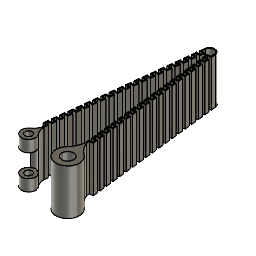
bones_v1 (Autodesk Fusion 360 design; units mm, degrees)
Autodesk Fusion 360 part; units mm, degrees
sketch "Sketch1" plane through (0, 0, 0) normal (0, 0, 1) x (1, 0, 0)
  circle A0 centre (68.7652, 38.9351) radius 1.9
  circle A1 centre (68.7652, 38.9351) radius 3.775
  line L0 (68.7652, 38.9351) -> (89.7652, 38.9351) construction
  circle A2 centre (89.7652, 38.9351) radius 3.175
  circle A3 centre (89.7652, 38.9351) radius 6.35
  line L1 (79.2652, 131.0925) -> (89.7652, 38.9351) construction
  line L2 (79.2652, 131.0925) -> (68.7652, 38.9351) construction
  line L3 (89.0463, 45.2443) -> (88.4803, 50.2122) construction
  line L4 (88.4803, 50.2122) -> (88.7287, 50.2405)
  line L5 (88.4803, 50.2122) -> (88.2319, 50.1839)
  line L6 (88.2319, 50.1839) -> (88.0055, 52.171)
  line L7 (88.7287, 50.2405) -> (88.5589, 51.7308)
  line L8 (88.0055, 52.171) -> (89.9927, 52.3974)
  line L9 (88.5589, 51.7308) -> (90.5461, 51.9573)
  line L10 (89.9927, 52.3974) -> (89.8229, 53.8878)
  line L11 (90.5461, 51.9573) -> (90.2631, 54.4412)
  line L12 (89.8229, 53.8878) -> (87.8357, 53.6614)
  line L13 (90.2631, 54.4412) -> (88.2759, 54.2148)
  line L14 (87.8357, 53.6614) -> (87.5527, 56.1453)
  line L15 (88.2759, 54.2148) -> (88.1061, 55.7051)
  line L16 (89.2261, 43.667) -> (93.3992, 44.1425) construction
  line L17 (89.2261, 43.667) -> (85.0529, 43.1916) construction
  arc A4 (85.0529, 43.1916) -> (88.2319, 50.1839) centre (75.649, 51.6858) ccw
  arc A5 (88.7287, 50.2405) -> (93.3992, 44.1425) centre (100.6513, 54.5345) ccw
  line L18 (88.1061, 55.7051) -> (90.0933, 55.9315)
  line L19 (87.5527, 56.1453) -> (89.5399, 56.3717)
  line L20 (89.5399, 56.3717) -> (89.3701, 57.8621)
  line L21 (90.0933, 55.9315) -> (89.8102, 58.4155)
  line L22 (89.8102, 58.4155) -> (87.8231, 58.1891)
  line L23 (89.3701, 57.8621) -> (87.3829, 57.6357)
  line L24 (87.3829, 57.6357) -> (87.0999, 60.1196)
  line L25 (87.8231, 58.1891) -> (87.6533, 59.6794)
  line L26 (87.6533, 59.6794) -> (89.6404, 59.9058)
  line L27 (87.0999, 60.1196) -> (89.0871, 60.346)
  line L28 (89.0871, 60.346) -> (88.9172, 61.8364)
  line L29 (89.6404, 59.9058) -> (89.3574, 62.3898)
  line L30 (88.9172, 61.8364) -> (86.9301, 61.61)
  line L31 (89.3574, 62.3898) -> (87.3703, 62.1634)
  line L32 (86.9301, 61.61) -> (86.6471, 64.0939)
  line L33 (87.3703, 62.1634) -> (87.2005, 63.6537)
  line L34 (87.2005, 63.6537) -> (89.1876, 63.8801)
  line L35 (86.6471, 64.0939) -> (88.6342, 64.3203)
  line L36 (88.6342, 64.3203) -> (88.4644, 65.8107)
  line L37 (89.1876, 63.8801) -> (88.9046, 66.364)
  line L38 (88.4644, 65.8107) -> (86.4773, 65.5843)
  line L39 (88.9046, 66.364) -> (86.9175, 66.1376)
  line L40 (86.4773, 65.5843) -> (86.1943, 68.0682)
  line L41 (86.9175, 66.1376) -> (86.7477, 67.628)
  line L42 (86.7477, 67.628) -> (88.7348, 67.8544)
  line L43 (86.1943, 68.0682) -> (88.1814, 68.2946)
  line L44 (88.1814, 68.2946) -> (88.0116, 69.7849)
  line L45 (88.7348, 67.8544) -> (88.4518, 70.3383)
  line L46 (88.0116, 69.7849) -> (86.0245, 69.5585)
  line L47 (88.4518, 70.3383) -> (86.4647, 70.1119)
  line L48 (86.0245, 69.5585) -> (85.7415, 72.0425)
  line L49 (86.4647, 70.1119) -> (86.2949, 71.6023)
  line L50 (86.2949, 71.6023) -> (88.282, 71.8287)
  line L51 (85.7415, 72.0425) -> (87.7286, 72.2689)
  line L52 (87.7286, 72.2689) -> (87.5588, 73.7592)
  line L53 (88.282, 71.8287) -> (87.999, 74.3126)
  line L54 (87.5588, 73.7592) -> (85.5717, 73.5328)
  line L55 (87.999, 74.3126) -> (86.0118, 74.0862)
  line L56 (85.5717, 73.5328) -> (85.2887, 76.0168)
  line L57 (86.0118, 74.0862) -> (85.842, 75.5766)
  line L58 (85.842, 75.5766) -> (87.8292, 75.803)
  line L59 (85.2887, 76.0168) -> (87.2758, 76.2432)
  line L60 (87.2758, 76.2432) -> (87.106, 77.7335)
  line L61 (87.8292, 75.803) -> (87.5462, 78.2869)
  line L62 (87.106, 77.7335) -> (85.1189, 77.5071)
  line L63 (87.5462, 78.2869) -> (85.559, 78.0605)
  line L64 (85.1189, 77.5071) -> (84.8358, 79.991)
  line L65 (85.559, 78.0605) -> (85.3892, 79.5509)
  line L66 (85.3892, 79.5509) -> (87.3764, 79.7773)
  line L67 (84.8358, 79.991) -> (86.823, 80.2175)
  line L68 (86.823, 80.2175) -> (86.6532, 81.7078)
  line L69 (87.3764, 79.7773) -> (87.0934, 82.2612)
  line L70 (86.6532, 81.7078) -> (84.666, 81.4814)
  line L71 (87.0934, 82.2612) -> (85.1062, 82.0348)
  line L72 (84.666, 81.4814) -> (84.383, 83.9653)
  line L73 (85.1062, 82.0348) -> (84.9364, 83.5251)
  line L74 (84.9364, 83.5251) -> (86.9236, 83.7516)
  line L75 (84.383, 83.9653) -> (86.3702, 84.1917)
  line L76 (86.3702, 84.1917) -> (86.2004, 85.6821)
  line L77 (86.9236, 83.7516) -> (86.6406, 86.2355)
  line L78 (86.2004, 85.6821) -> (84.2132, 85.4557)
  line L79 (86.6406, 86.2355) -> (84.6534, 86.0091)
  line L80 (84.2132, 85.4557) -> (83.9302, 87.9396)
  line L81 (84.6534, 86.0091) -> (84.4836, 87.4994)
  line L82 (84.4836, 87.4994) -> (86.4707, 87.7258)
  line L83 (83.9302, 87.9396) -> (85.9174, 88.166)
  line L84 (85.9174, 88.166) -> (85.7476, 89.6564)
  line L85 (86.4707, 87.7258) -> (86.1877, 90.2098)
  line L86 (85.7476, 89.6564) -> (83.7604, 89.43)
  line L87 (86.1877, 90.2098) -> (84.2006, 89.9834)
  line L88 (83.7604, 89.43) -> (83.4774, 91.9139)
  line L89 (84.2006, 89.9834) -> (84.0308, 91.4737)
  line L90 (84.0308, 91.4737) -> (86.0179, 91.7001)
  line L91 (83.4774, 91.9139) -> (85.4645, 92.1403)
  line L92 (85.4645, 92.1403) -> (85.2947, 93.6307)
  line L93 (86.0179, 91.7001) -> (85.7349, 94.1841)
  line L94 (85.2947, 93.6307) -> (83.3076, 93.4043)
  line L95 (85.7349, 94.1841) -> (83.7478, 93.9577)
  line L96 (83.3076, 93.4043) -> (83.0246, 95.8882)
  line L97 (83.7478, 93.9577) -> (83.578, 95.448)
  line L98 (83.578, 95.448) -> (85.5651, 95.6744)
  line L99 (83.0246, 95.8882) -> (85.0117, 96.1146)
  line L100 (85.0117, 96.1146) -> (84.8419, 97.605)
  line L101 (85.5651, 95.6744) -> (85.2821, 98.1583)
  line L102 (84.8419, 97.605) -> (82.8548, 97.3786)
  line L103 (85.2821, 98.1583) -> (83.295, 97.9319)
  line L104 (82.8548, 97.3786) -> (82.5718, 99.8625)
  line L105 (83.295, 97.9319) -> (83.1252, 99.4223)
  line L106 (83.1252, 99.4223) -> (85.1123, 99.6487)
  line L107 (82.5718, 99.8625) -> (84.5589, 100.0889)
  line L108 (84.5589, 100.0889) -> (84.3891, 101.5792)
  line L109 (85.1123, 99.6487) -> (84.8293, 102.1326)
  line L110 (84.3891, 101.5792) -> (82.402, 101.3528)
  line L111 (84.8293, 102.1326) -> (82.8422, 101.9062)
  line L112 (82.402, 101.3528) -> (82.119, 103.8368)
  line L113 (82.8422, 101.9062) -> (82.6724, 103.3966)
  line L114 (82.6724, 103.3966) -> (84.6595, 103.623)
  line L115 (82.119, 103.8368) -> (84.1061, 104.0632)
  line L116 (84.1061, 104.0632) -> (83.9363, 105.5535)
  line L117 (84.6595, 103.623) -> (84.3765, 106.1069)
  line L118 (83.9363, 105.5535) -> (81.9492, 105.3271)
  line L119 (84.3765, 106.1069) -> (82.3893, 105.8805)
  line L120 (81.9492, 105.3271) -> (81.6662, 107.8111)
  line L121 (82.3893, 105.8805) -> (82.2195, 107.3709)
  line L122 (82.2195, 107.3709) -> (84.2067, 107.5973)
  line L123 (81.6662, 107.8111) -> (83.6533, 108.0375)
  line L124 (83.6533, 108.0375) -> (83.4835, 109.5278)
  line L125 (84.2067, 107.5973) -> (83.9237, 110.0812)
  line L126 (83.4835, 109.5278) -> (81.4963, 109.3014)
  line L127 (83.9237, 110.0812) -> (81.9365, 109.8548)
  line L128 (81.4963, 109.3014) -> (81.2133, 111.7853)
  line L129 (81.9365, 109.8548) -> (81.7667, 111.3452)
  line L130 (81.7667, 111.3452) -> (83.7539, 111.5716)
  line L131 (81.2133, 111.7853) -> (83.2005, 112.0118)
  line L132 (83.2005, 112.0118) -> (83.0307, 113.5021)
  line L133 (83.7539, 111.5716) -> (83.4709, 114.0555)
  line L134 (83.0307, 113.5021) -> (81.0435, 113.2757)
  line L135 (83.4709, 114.0555) -> (81.4837, 113.8291)
  line L136 (81.0435, 113.2757) -> (80.7605, 115.7596)
  line L137 (81.4837, 113.8291) -> (81.3139, 115.3194)
  line L138 (88.5589, 51.7308) -> (90.5461, 51.9573)
  line L139 (88.0055, 52.171) -> (89.9927, 52.3974)
  line L140 (89.9927, 52.3974) -> (89.8229, 53.8878)
  line L141 (90.5461, 51.9573) -> (90.2631, 54.4412)
  line L142 (89.8229, 53.8878) -> (87.8357, 53.6614)
  line L143 (90.2631, 54.4412) -> (88.2759, 54.2148)
  line L144 (87.8357, 53.6614) -> (87.5527, 56.1453)
  line L145 (88.2759, 54.2148) -> (88.1061, 55.7051)
  line L146 (88.1061, 55.7051) -> (90.0933, 55.9315)
  line L147 (87.5527, 56.1453) -> (89.5399, 56.3717)
  line L148 (89.5399, 56.3717) -> (89.3701, 57.8621)
  line L149 (90.0933, 55.9315) -> (89.8102, 58.4155)
  line L150 (89.3701, 57.8621) -> (87.3829, 57.6357)
  line L151 (89.8102, 58.4155) -> (87.8231, 58.1891)
  line L152 (87.3829, 57.6357) -> (87.0999, 60.1196)
  line L153 (87.8231, 58.1891) -> (87.6533, 59.6794)
  line L154 (81.3139, 115.3194) -> (83.3011, 115.5459)
  line L155 (80.7605, 115.7596) -> (82.7477, 115.986)
  line L156 (82.7477, 115.986) -> (82.5779, 117.4764)
  line L157 (83.3011, 115.5459) -> (83.0181, 118.0298)
  line L158 (82.5779, 117.4764) -> (80.5907, 117.25)
  line L159 (83.0181, 118.0298) -> (81.0309, 117.8034)
  line L160 (80.5907, 117.25) -> (80.3077, 119.7339)
  line L161 (81.0309, 117.8034) -> (80.8611, 119.2937)
  line L162 (80.8611, 119.2937) -> (82.8482, 119.5201)
  line L163 (80.3077, 119.7339) -> (82.2949, 119.9603)
  line L164 (82.2949, 119.9603) -> (82.1251, 121.4507)
  line L165 (82.8482, 119.5201) -> (82.5652, 122.0041)
  line L166 (82.1251, 121.4507) -> (80.1379, 121.2243)
  line L167 (82.5652, 122.0041) -> (80.5781, 121.7777)
  line L168 (80.1379, 121.2243) -> (79.8549, 123.7082)
  line L169 (80.5781, 121.7777) -> (80.4083, 123.268)
  line L170 (80.4083, 123.268) -> (82.3954, 123.4944)
  line L171 (79.8549, 123.7082) -> (81.842, 123.9346)
  line L172 (81.842, 123.9346) -> (81.6722, 125.425)
  line L173 (82.3954, 123.4944) -> (82.1124, 125.9784)
  line L174 (79.2652, 131.0925) -> (79.2652, 38.9351) construction
  line L175 (80.8611, 119.2937) -> (82.8482, 119.5201)
  line L176 (80.3077, 119.7339) -> (82.2949, 119.9603)
  line L177 (82.2949, 119.9603) -> (82.1251, 121.4507)
  line L178 (82.8482, 119.5201) -> (82.5652, 122.0041)
  line L179 (76.141, 105.8805) -> (76.3108, 107.3709)
  line L180 (75.0469, 109.5278) -> (77.034, 109.3014)
  line L181 (74.6067, 110.0812) -> (76.5938, 109.8548)
  line L182 (74.1539, 106.1069) -> (76.141, 105.8805)
  line L183 (73.7011, 102.1326) -> (75.6882, 101.9062)
  line L184 (76.1284, 101.3528) -> (76.4114, 103.8368)
  line L185 (74.5941, 105.5535) -> (76.5812, 105.3271)
  line L186 (74.3237, 107.5973) -> (74.6067, 110.0812)
  line L187 (74.1413, 101.5792) -> (76.1284, 101.3528)
  line L188 (76.5812, 105.3271) -> (76.8642, 107.8111)
  line L189 (73.4181, 99.6487) -> (73.7011, 102.1326)
  line L190 (75.6821, 119.5201) -> (75.9651, 122.0041)
  line L191 (76.6883, 123.9346) -> (76.8581, 125.425)
  line L192 (76.2355, 119.9603) -> (76.4053, 121.4507)
  line L193 (77.9523, 121.7777) -> (78.1221, 123.268)
  line L194 (77.9397, 117.25) -> (78.2227, 119.7339)
  line L195 (77.4868, 113.2757) -> (77.7699, 115.7596)
  line L196 (78.6755, 123.7082) -> (76.6883, 123.9346)
  line L197 (75.5123, 118.0298) -> (77.4995, 117.8034)
  line L198 (70.6946, 53.6614) -> (70.9777, 56.1453)
  line L199 (75.4997, 113.5021) -> (77.4868, 113.2757)
  line L200 (77.0467, 113.8291) -> (77.2165, 115.3194)
  line L201 (78.1221, 123.268) -> (76.1349, 123.4944)
  line L202 (70.6946, 53.6614) -> (70.9777, 56.1453)
  line L203 (74.3172, 85.4557) -> (74.6002, 87.9396)
  line L204 (77.6693, 119.2937) -> (75.6821, 119.5201)
  line L205 (78.3925, 121.2243) -> (78.6755, 123.7082)
  line L206 (75.9651, 122.0041) -> (77.9523, 121.7777)
  line L207 (75.9525, 117.4764) -> (77.9397, 117.25)
  line L208 (70.2545, 54.2148) -> (70.4243, 55.7051)
  line L209 (78.2227, 119.7339) -> (76.2355, 119.9603)
  line L210 (76.4053, 121.4507) -> (78.3925, 121.2243)
  line L211 (70.2545, 54.2148) -> (70.4243, 55.7051)
  line L212 (75.2293, 115.5459) -> (75.5123, 118.0298)
  line L213 (75.0595, 114.0555) -> (77.0467, 113.8291)
  line L214 (76.2355, 119.9603) -> (76.4053, 121.4507)
  line L215 (68.4371, 55.9315) -> (68.7201, 58.4155)
  line L216 (69.9715, 51.7308) -> (67.9843, 51.9573)
  line L217 (77.2165, 115.3194) -> (75.2293, 115.5459)
  line L218 (77.317, 111.7853) -> (75.3299, 112.0118)
  line L219 (70.5248, 52.171) -> (68.5377, 52.3974)
  line L220 (68.7075, 53.8878) -> (70.6946, 53.6614)
  line L221 (75.3299, 112.0118) -> (75.4997, 113.5021)
  line L222 (70.5248, 52.171) -> (68.5377, 52.3974)
  line L223 (76.7636, 111.3452) -> (74.7765, 111.5716)
  line L224 (77.7699, 115.7596) -> (75.7827, 115.986)
  line L225 (68.2673, 54.4412) -> (70.2545, 54.2148)
  line L226 (74.7765, 111.5716) -> (75.0595, 114.0555)
  line L227 (73.5186, 96.1146) -> (73.6884, 97.605)
  line L228 (75.6821, 119.5201) -> (75.9651, 122.0041)
  line L229 (75.7827, 115.986) -> (75.9525, 117.4764)
  line L230 (72.9653, 95.6744) -> (73.2483, 98.1583)
  line L231 (77.034, 109.3014) -> (77.317, 111.7853)
  line L232 (76.5938, 109.8548) -> (76.7636, 111.3452)
  line L233 (68.7075, 53.8878) -> (70.6946, 53.6614)
  line L234 (78.2227, 119.7339) -> (76.2355, 119.9603)
  line L235 (77.4995, 117.8034) -> (77.6693, 119.2937)
  line L236 (68.5377, 52.3974) -> (68.7075, 53.8878)
  line L237 (67.9843, 51.9573) -> (68.2673, 54.4412)
  line L238 (68.2673, 54.4412) -> (70.2545, 54.2148)
  line L239 (77.6693, 119.2937) -> (75.6821, 119.5201)
  line L240 (67.9843, 51.9573) -> (68.2673, 54.4412)
  line L241 (68.5377, 52.3974) -> (68.7075, 53.8878)
  line L242 (76.1349, 123.4944) -> (76.418, 125.9784)
  line L243 (69.9715, 51.7308) -> (67.9843, 51.9573)
  line L244 (68.9905, 56.3717) -> (69.1603, 57.8621)
  line L245 (74.1473, 83.9653) -> (72.1602, 84.1917)
  line L246 (73.594, 83.5251) -> (71.6068, 83.7516)
  line L247 (68.7201, 58.4155) -> (70.7073, 58.1891)
  line L248 (73.2417, 76.0168) -> (71.2546, 76.2432)
  line L249 (69.1603, 57.8621) -> (71.1475, 57.6357)
  line L250 (70.4243, 55.7051) -> (68.4371, 55.9315)
  line L251 (70.9777, 56.1453) -> (68.9905, 56.3717)
  line L252 (71.154, 79.7773) -> (71.437, 82.2612)
  line L253 (73.4115, 77.5071) -> (73.6945, 79.991)
  line L254 (68.9905, 56.3717) -> (69.1603, 57.8621)
  line L255 (69.4433, 60.346) -> (69.6131, 61.8364)
  line L256 (70.0659, 65.8107) -> (72.0531, 65.5843)
  line L257 (75.5058, 95.8882) -> (73.5186, 96.1146)
  line L258 (71.6003, 61.61) -> (71.8833, 64.0939)
  line L259 (72.7954, 94.1841) -> (74.7826, 93.9577)
  line L260 (74.9524, 95.448) -> (72.9653, 95.6744)
  line L261 (74.77, 89.43) -> (75.053, 91.9139)
  line L262 (71.8833, 64.0939) -> (69.8961, 64.3203)
  line L263 (73.2356, 93.6307) -> (75.2228, 93.4043)
  line L264 (72.2355, 71.6023) -> (70.2484, 71.8287)
  line L265 (70.349, 68.2946) -> (70.5188, 69.7849)
  line L266 (74.6002, 87.9396) -> (72.613, 88.166)
  line L267 (72.5124, 91.7001) -> (72.7954, 94.1841)
  line L268 (70.5188, 69.7849) -> (72.5059, 69.5585)
  line L269 (74.3298, 89.9834) -> (74.4996, 91.4737)
  line L270 (75.2228, 93.4043) -> (75.5058, 95.8882)
  line L271 (69.7956, 67.8544) -> (70.0786, 70.3383)
  line L272 (69.8961, 64.3203) -> (70.0659, 65.8107)
  line L273 (74.4996, 91.4737) -> (72.5124, 91.7001)
  line L274 (72.3426, 90.2098) -> (74.3298, 89.9834)
  line L275 (71.1601, 62.1634) -> (71.3299, 63.6537)
  line L276 (70.8771, 59.6794) -> (68.8899, 59.9058)
  line L277 (72.5059, 69.5585) -> (72.7889, 72.0425)
  line L278 (71.7827, 67.628) -> (69.7956, 67.8544)
  line L279 (69.6258, 66.364) -> (71.6129, 66.1376)
  line L280 (74.8771, 108.0375) -> (75.0469, 109.5278)
  line L281 (69.6131, 61.8364) -> (71.6003, 61.61)
  line L282 (73.877, 86.0091) -> (74.0468, 87.4994)
  line L283 (72.6883, 75.5766) -> (70.7012, 75.803)
  line L284 (70.7073, 58.1891) -> (70.8771, 59.6794)
  line L285 (70.9842, 78.2869) -> (72.9713, 78.0605)
  line L286 (71.1475, 57.6357) -> (71.4305, 60.1196)
  line L287 (70.7073, 58.1891) -> (70.8771, 59.6794)
  line L288 (71.1475, 57.6357) -> (71.4305, 60.1196)
  line L289 (70.8018, 72.2689) -> (70.9716, 73.7592)
  line L290 (73.4242, 82.0348) -> (73.594, 83.5251)
  line L291 (70.2484, 71.8287) -> (70.5314, 74.3126)
  line L292 (73.6945, 79.991) -> (71.7074, 80.2175)
  line L293 (71.8898, 86.2355) -> (73.877, 86.0091)
  line L294 (75.858, 103.3966) -> (73.8709, 103.623)
  line L295 (76.4114, 103.8368) -> (74.4243, 104.0632)
  line L296 (74.4243, 104.0632) -> (74.5941, 105.5535)
  line L297 (73.2483, 98.1583) -> (75.2354, 97.9319)
  line L298 (76.8642, 107.8111) -> (74.8771, 108.0375)
  line L299 (75.4052, 99.4223) -> (73.4181, 99.6487)
  line L300 (75.6882, 101.9062) -> (75.858, 103.3966)
  line L301 (73.6884, 97.605) -> (75.6756, 97.3786)
  line L302 (76.3108, 107.3709) -> (74.3237, 107.5973)
  line L303 (75.2354, 97.9319) -> (75.4052, 99.4223)
  line L304 (73.8709, 103.623) -> (74.1539, 106.1069)
  line L305 (75.9586, 99.8625) -> (73.9715, 100.0889)
  line L306 (75.6756, 97.3786) -> (75.9586, 99.8625)
  line L307 (73.9715, 100.0889) -> (74.1413, 101.5792)
  line L308 (71.8772, 81.7078) -> (73.8643, 81.4814)
  line L309 (68.4371, 55.9315) -> (68.7201, 58.4155)
  line L310 (71.4244, 77.7335) -> (73.4115, 77.5071)
  line L311 (70.9777, 56.1453) -> (68.9905, 56.3717)
  line L312 (70.5314, 74.3126) -> (72.5185, 74.0862)
  line L313 (71.6068, 83.7516) -> (71.8898, 86.2355)
  line L314 (70.4243, 55.7051) -> (68.4371, 55.9315)
  line L315 (70.7012, 75.803) -> (70.9842, 78.2869)
  line L316 (72.5185, 74.0862) -> (72.6883, 75.5766)
  line L317 (69.1603, 57.8621) -> (71.1475, 57.6357)
  line L318 (71.7074, 80.2175) -> (71.8772, 81.7078)
  line L319 (72.9713, 78.0605) -> (73.1411, 79.5509)
  line L320 (72.33, 85.6821) -> (74.3172, 85.4557)
  line L321 (68.7201, 58.4155) -> (70.7073, 58.1891)
  line L322 (71.437, 82.2612) -> (73.4242, 82.0348)
  line L323 (70.9716, 73.7592) -> (72.9587, 73.5328)
  line L324 (75.053, 91.9139) -> (73.0658, 92.1403)
  line L325 (73.8643, 81.4814) -> (74.1473, 83.9653)
  line L326 (73.1411, 79.5509) -> (71.154, 79.7773)
  line L327 (72.9587, 73.5328) -> (73.2417, 76.0168)
  line L328 (72.1602, 84.1917) -> (72.33, 85.6821)
  line L329 (71.2546, 76.2432) -> (71.4244, 77.7335)
  line L330 (72.0657, 70.1119) -> (72.2355, 71.6023)
  line L331 (71.6129, 66.1376) -> (71.7827, 67.628)
  line L332 (71.3299, 63.6537) -> (69.3428, 63.8801)
  line L333 (70.0786, 70.3383) -> (72.0657, 70.1119)
  line L334 (72.3361, 68.0682) -> (70.349, 68.2946)
  line L335 (74.0468, 87.4994) -> (72.0596, 87.7258)
  line L336 (69.3428, 63.8801) -> (69.6258, 66.364)
  line L337 (73.0658, 92.1403) -> (73.2356, 93.6307)
  line L338 (72.7828, 89.6564) -> (74.77, 89.43)
  line L339 (72.0596, 87.7258) -> (72.3426, 90.2098)
  line L340 (69.1729, 62.3898) -> (71.1601, 62.1634)
  line L341 (72.0531, 65.5843) -> (72.3361, 68.0682)
  line L342 (74.7826, 93.9577) -> (74.9524, 95.448)
  line L343 (71.4305, 60.1196) -> (69.4433, 60.346)
  line L344 (72.613, 88.166) -> (72.7828, 89.6564)
  line L345 (68.8899, 59.9058) -> (69.1729, 62.3898)
  line L346 (72.7889, 72.0425) -> (70.8018, 72.2689)
  line L347 (69.8017, 50.2405) -> (69.9715, 51.7308)
  line L348 (70.2418, 49.6871) -> (70.5248, 52.171)
  line L349 (68.2547, 49.9135) -> (70.2418, 49.6871)
  line L350 (67.8145, 50.4669) -> (69.8017, 50.2405)
  line L351 (67.5315, 47.983) -> (67.8145, 50.4669)
  line L352 (68.0849, 48.4232) -> (68.2547, 49.9135)
  line L353 (70.072, 48.1967) -> (68.0849, 48.4232)
  line L354 (69.5186, 47.7566) -> (67.5315, 47.983)
  line L355 (70.072, 48.1967) -> (69.8456, 46.2096)
  line L356 (69.5186, 47.7566) -> (69.3488, 46.2662)
  line L357 (69.8456, 46.2096) -> (69.3488, 46.2662)
  line L358 (69.0864, 41.7544) -> (71.5602, 41.4726) construction
  line L359 (69.0864, 41.7544) -> (66.6126, 42.0363) construction
  arc A6 (66.6126, 42.0363) -> (69.3488, 46.2662) centre (62.8331, 47.4811) ccw
  arc A7 (69.8456, 46.2096) -> (71.5602, 41.4726) centre (76.4676, 45.9276) ccw
  line L360 (76.8581, 125.425) -> (76.9147, 125.9218)
  line L361 (81.6722, 125.425) -> (81.6156, 125.9218)
  arc A8 (82.1124, 125.9784) -> (76.418, 125.9784) centre (79.2652, 125.654) ccw
  arc A9 (81.6156, 125.9218) -> (76.9147, 125.9218) centre (79.2652, 125.654) ccw
  point P0 (79.2652, 131.0925)
  dimension "d1" = 3.8
  dimension "d2" = 7.55
  dimension "d3" = 21
  dimension "d4" = 6.35
  dimension "d5" = 12.7
  dimension "d8" = 83.5
  dimension "d9" = 83.5
  constraint concentric A0 A1
  constraint coincident A0.centre A1.centre
  constraint horizontal L0
  constraint coincident L0.end A2.centre
  constraint concentric A2 A3
  constraint coincident P0 L1.start
  constraint coincident L1 L3.start
  constraint coincident A3 L3.start
  constraint parallel L1 L3
  constraint perpendicular L3 L4
  constraint perpendicular L1 L5
  constraint perpendicular L5 L6
  constraint perpendicular L4 L7
  constraint perpendicular L6 L8
  constraint perpendicular L7 L9
  constraint perpendicular L8 L10
  constraint perpendicular L9 L11
  constraint perpendicular L1 L12
  constraint perpendicular L11 L13
  constraint perpendicular L12 L14
  constraint perpendicular L13 L15
  constraint coincident A3 L16.end
  constraint perpendicular L1 L16
  constraint coincident A3 L17.end
  constraint perpendicular L1 L17
  constraint tangent A3 A4
  constraint tangent A3 A5
  constraint perpendicular L19 L20
  constraint perpendicular L18 L21
  constraint perpendicular L21 L22
  constraint perpendicular L23 L24
  constraint perpendicular L22 L25
  constraint perpendicular L27 L28
  constraint perpendicular L26 L29
  constraint perpendicular L29 L31
  constraint perpendicular L30 L32
  constraint perpendicular L31 L33
  constraint perpendicular L35 L36
  constraint perpendicular L34 L37
  constraint perpendicular L37 L39
  constraint perpendicular L38 L40
  constraint perpendicular L39 L41
  constraint perpendicular L43 L44
  constraint perpendicular L42 L45
  constraint perpendicular L45 L47
  constraint perpendicular L46 L48
  constraint perpendicular L47 L49
  constraint perpendicular L51 L52
  constraint perpendicular L50 L53
  constraint perpendicular L53 L55
  constraint perpendicular L54 L56
  constraint perpendicular L55 L57
  constraint perpendicular L59 L60
  constraint perpendicular L58 L61
  constraint perpendicular L61 L63
  constraint perpendicular L62 L64
  constraint perpendicular L63 L65
  constraint perpendicular L67 L68
  constraint perpendicular L66 L69
  constraint perpendicular L69 L71
  constraint perpendicular L70 L72
  constraint perpendicular L71 L73
  constraint perpendicular L75 L76
  constraint perpendicular L74 L77
  constraint perpendicular L77 L79
  constraint perpendicular L78 L80
  constraint perpendicular L79 L81
  constraint perpendicular L83 L84
  constraint perpendicular L82 L85
  constraint perpendicular L85 L87
  constraint perpendicular L86 L88
  constraint perpendicular L87 L89
  constraint perpendicular L91 L92
  constraint perpendicular L90 L93
  constraint perpendicular L93 L95
  constraint perpendicular L94 L96
  constraint perpendicular L95 L97
  constraint perpendicular L99 L100
  constraint perpendicular L98 L101
  constraint perpendicular L101 L103
  constraint perpendicular L102 L104
  constraint perpendicular L103 L105
  constraint perpendicular L107 L108
  constraint perpendicular L106 L109
  constraint perpendicular L109 L111
  constraint perpendicular L110 L112
  constraint perpendicular L111 L113
  constraint perpendicular L115 L116
  constraint perpendicular L114 L117
  constraint perpendicular L117 L119
  constraint perpendicular L118 L120
  constraint perpendicular L119 L121
  constraint perpendicular L123 L124
  constraint perpendicular L122 L125
  constraint perpendicular L125 L127
  constraint perpendicular L126 L128
  constraint perpendicular L127 L129
  constraint perpendicular L131 L132
  constraint perpendicular L130 L133
  constraint perpendicular L133 L135
  constraint perpendicular L134 L136
  constraint perpendicular L135 L137
  constraint perpendicular L139 L140
  constraint perpendicular L138 L141
  constraint perpendicular L141 L143
  constraint perpendicular L142 L144
  constraint perpendicular L143 L145
  constraint perpendicular L147 L148
  constraint perpendicular L146 L149
  constraint perpendicular L149 L151
  constraint perpendicular L150 L152
  constraint perpendicular L151 L153
  constraint perpendicular L155 L156
  constraint perpendicular L154 L157
  constraint perpendicular L157 L159
  constraint perpendicular L158 L160
  constraint perpendicular L159 L161
  constraint perpendicular L163 L164
  constraint perpendicular L162 L165
  constraint perpendicular L165 L167
  constraint perpendicular L166 L168
  constraint perpendicular L167 L169
  constraint perpendicular L171 L172
  constraint perpendicular L170 L173
  constraint midpoint L0 L174.end
  constraint perpendicular L176 L177
  constraint perpendicular L175 L178
  constraint symmetric L6.end L174 L219.start
  constraint symmetric L7.end L174 L216.start
  constraint symmetric L8.end L174 L219.end
  constraint symmetric L9.end L174 L216.end
  constraint symmetric L10.end L174 L220.start
  constraint symmetric L11.end L174 L225.start
  constraint symmetric L12.end L174 L198.start
  constraint symmetric L13.end L174 L208.start
  constraint symmetric L14.end L174 L198.end
  constraint symmetric L15.end L174 L208.end
  constraint symmetric L19.end L174 L244.start
  constraint symmetric L20.end L174 L244.end
  constraint symmetric L18.end L174 L215.start
  constraint symmetric L22.end L174 L247.end
  constraint symmetric L21.end L174 L215.end
  constraint symmetric L23.end L174 L249.end
  constraint symmetric L24.end L174 L286.end
  constraint symmetric L25.end L174 L276.start
  constraint symmetric L27.end L174 L255.start
  constraint symmetric L28.end L174 L255.end
  constraint symmetric L26.end L174 L276.end
  constraint symmetric L31.end L174 L275.start
  constraint symmetric L29.end L174 L340.start
  constraint symmetric L30.end L174 L258.start
  constraint symmetric L32.end L174 L258.end
  constraint symmetric L39.end L174 L279.end
  constraint symmetric L36.end L174 L256.start
  constraint symmetric L38.end L174 L256.end
  constraint symmetric L41.end L174 L278.start
  constraint symmetric L37.end L174 L279.start
  constraint symmetric L35.end L174 L262.end
  constraint symmetric L34.end L174 L332.end
  constraint symmetric L40.end L174 L334.start
  constraint symmetric L33.end L174 L275.end
  constraint symmetric L43.end L174 L265.start
  constraint symmetric L44.end L174 L265.end
  constraint symmetric L42.end L174 L271.start
  constraint symmetric L47.end L174 L330.start
  constraint symmetric L45.end L174 L271.end
  constraint symmetric L46.end L174 L268.end
  constraint symmetric L48.end L174 L277.end
  constraint symmetric L55.end L174 L312.end
  constraint symmetric L52.end L174 L289.end
  constraint symmetric L54.end L174 L323.end
  constraint symmetric L57.end L174 L283.start
  constraint symmetric L53.end L174 L291.end
  constraint symmetric L51.end L174 L289.start
  constraint symmetric L50.end L174 L264.end
  constraint symmetric L56.end L174 L248.start
  constraint symmetric L49.end L174 L264.start
  constraint symmetric L59.end L174 L248.end
  constraint symmetric L60.end L174 L310.start
  constraint symmetric L58.end L174 L283.end
  constraint symmetric L63.end L174 L285.end
  constraint symmetric L61.end L174 L285.start
  constraint symmetric L62.end L174 L253.start
  constraint symmetric L64.end L174 L253.end
  constraint symmetric L71.end L174 L290.start
  constraint symmetric L68.end L174 L308.start
  constraint symmetric L70.end L174 L308.end
  constraint symmetric L73.end L174 L246.start
  constraint symmetric L69.end L174 L252.end
  constraint symmetric L67.end L174 L292.end
  constraint symmetric L66.end L174 L252.start
  constraint symmetric L72.end L174 L245.start
  constraint symmetric L65.end L174 L319.end
  constraint symmetric L75.end L174 L245.end
  constraint symmetric L76.end L174 L320.start
  constraint symmetric L74.end L174 L246.end
  constraint symmetric L79.end L174 L282.start
  constraint symmetric L77.end L174 L293.start
  constraint symmetric L78.end L174 L203.start
  constraint symmetric L80.end L174 L203.end
  constraint symmetric L87.end L174 L269.start
  constraint symmetric L84.end L174 L338.start
  constraint symmetric L86.end L174 L261.start
  constraint symmetric L89.end L174 L269.end
  constraint symmetric L85.end L174 L274.start
  constraint symmetric L83.end L174 L266.end
  constraint symmetric L82.end L174 L335.end
  constraint symmetric L88.end L174 L261.end
  constraint symmetric L81.end L174 L282.end
  constraint symmetric L91.end L174 L324.end
  constraint symmetric L92.end L174 L263.start
  constraint symmetric L90.end L174 L267.start
  constraint symmetric L95.end L174 L259.end
  constraint symmetric L93.end L174 L259.start
  constraint symmetric L94.end L174 L263.end
  constraint symmetric L96.end L174 L257.start
  constraint symmetric L103.end L174 L297.end
  constraint symmetric L100.end L174 L227.end
  constraint symmetric L102.end L174 L301.end
  constraint symmetric L105.end L174 L299.start
  constraint symmetric L101.end L174 L230.end
  constraint symmetric L99.end L174 L227.start
  constraint symmetric L98.end L174 L230.start
  constraint symmetric L104.end L174 L305.start
  constraint symmetric L97.end L174 L260.start
  constraint symmetric L107.end L174 L305.end
  constraint symmetric L108.end L174 L187.start
  constraint symmetric L106.end L174 L189.start
  constraint symmetric L111.end L174 L183.end
  constraint symmetric L109.end L174 L183.start
  constraint symmetric L110.end L174 L184.start
  constraint symmetric L112.end L174 L184.end
  constraint symmetric L119.end L174 L179.start
  constraint symmetric L116.end L174 L185.start
  constraint symmetric L118.end L174 L185.end
  constraint symmetric L121.end L174 L179.end
  constraint symmetric L117.end L174 L182.start
  constraint symmetric L115.end L174 L295.end
  constraint symmetric L114.end L174 L294.end
  constraint symmetric L120.end L174 L188.end
  constraint symmetric L113.end L174 L294.start
  constraint symmetric L123.end L174 L280.start
  constraint symmetric L124.end L174 L180.start
  constraint symmetric L122.end L174 L186.start
  constraint symmetric L127.end L174 L181.end
  constraint symmetric L125.end L174 L181.start
  constraint symmetric L126.end L174 L180.end
  constraint symmetric L128.end L174 L218.start
  constraint symmetric L135.end L174 L200.start
  constraint symmetric L132.end L174 L199.start
  constraint symmetric L134.end L174 L195.start
  constraint symmetric L137.end L174 L200.end
  constraint symmetric L133.end L174 L213.start
  constraint symmetric L131.end L174 L218.end
  constraint symmetric L130.end L174 L223.end
  constraint symmetric L136.end L174 L195.end
  constraint symmetric L129.end L174 L223.start
  constraint symmetric L155.end L174 L224.end
  constraint symmetric L156.end L174 L207.start
  constraint symmetric L154.end L174 L212.start
  constraint symmetric L159.end L174 L197.end
  constraint symmetric L157.end L174 L197.start
  constraint symmetric L158.end L174 L194.start
  constraint symmetric L160.end L174 L194.end
  constraint symmetric L167.end L174 L193.start
  constraint symmetric L164.end L174 L192.end
  constraint symmetric L166.end L174 L205.start
  constraint symmetric L169.end L174 L193.end
  constraint symmetric L165.end L174 L190.end
  constraint symmetric L163.end L174 L192.start
  constraint symmetric L162.end L174 L190.start
  constraint symmetric L168.end L174 L196.start
  constraint symmetric L161.end L174 L204.start
  constraint symmetric L172.end L174 L191.end
  constraint symmetric L170.end L174 L201.end
  constraint symmetric L171.end L174 L191.start
  constraint symmetric L173.end L174 L242.end
  constraint symmetric L174 L164.end L192.end
  constraint symmetric L174 L162.end L190.start
  constraint symmetric L174 L161.end L204.start
  constraint symmetric L174 L160.end L194.end
  constraint symmetric L174 L163.end L192.start
  constraint symmetric L174 L165.end L190.end
  constraint perpendicular L353 L355
  constraint perpendicular L354 L356
  constraint perpendicular L356 L357
  constraint coincident A1 L358.end
  constraint perpendicular L2 L358
  constraint coincident A1 L359.end
  constraint perpendicular L2 L359
  constraint tangent A1 A6
  constraint tangent A1 A7
  constraint parallel L191 L360
  constraint parallel L172 L361
  constraint tangent L173 A8
  constraint tangent L242 A8
  constraint tangent L361 A9
  measures "d1" diameter of A0
  measures "d2" diameter of A1
  measures "d3" distance of A0.centre L0.end
  measures "d4" diameter of A2
  measures "d5" diameter of A3
  measures "d8" angle of L0 L2
  measures "d9" angle of L0 L1
extrude "Extrude1" add sketch "Sketch1" along normal blind 24.5
hole "Hole1" at (68.7652, 38.9351, 0) direction (0, 0, 1) diameter 7.55 depth 18.25 tip angle 180
extrude "Extrude2" add sketch "Sketch1" along normal blind 6.25 contours A1
